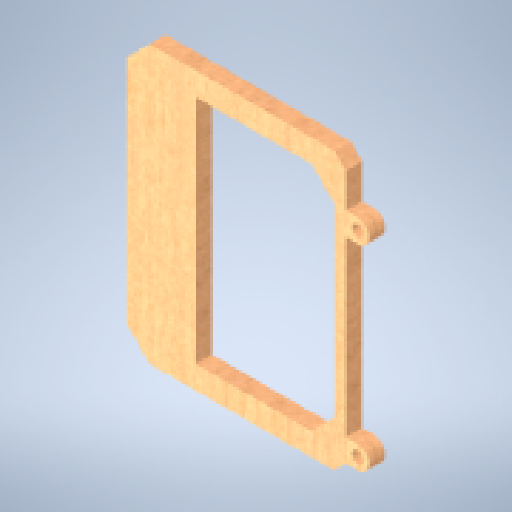
# Autodesk Inventor part: Tapa
Saved by Autodesk Inventor 2023.1 (Build 271208000, 208)
## iProperties
Created: 2022-10-30
Part Number: Tapa
Material: MDF Medium Density Fiberboard
Document SubType Name: Modeling
Designer: Daniel Peña
Density: 0.8 g/cm^3
Appearance: Cherry - Natural Low Gloss
Author: Daniel Peña
Autodesk Inventor part; units mm, degrees
ref_plane "YZ Plane" through (0, 0, 0) normal (1, 0, 0) x (0, 1, 0)
ref_plane "XZ Plane" through (0, 0, 0) normal (0, 1, 0) x (-1, 0, 0)
ref_plane "XY Plane" through (0, 0, 0) normal (0, 0, 1) x (1, 0, 0)
sketch "Sketch1" plane through (0, 0, 0) normal (0, 0, 1) x (1, 0, 0)
  circle A0 centre (47.5, -35) radius 2.5 projected
  circle A1 centre (47.5, 50) radius 2.5 projected
  circle A2 centre (47.5, 35) radius 2.5 projected
  circle A3 centre (47.5, -50) radius 2.5 projected
  line L0 (50, -65) -> (52.5, -62.5) projected
  line L1 (52.5, -62.5) -> (52.5, -15) projected
  line L2 (52.5, -15) -> (37.5, -15) projected
  line L3 (37.5, -15) -> (37.5, -40) projected
  line L4 (37.5, -40) -> (27.5, -50) projected
  line L5 (27.5, -50) -> (-22.5, -50) projected
  line L6 (-22.5, -50) -> (-22.5, 50) projected
  line L7 (-22.5, 50) -> (27.5, 50) projected
  line L8 (27.5, 50) -> (37.5, 40) projected
  line L9 (37.5, 40) -> (37.5, 15) projected
  line L10 (37.5, 15) -> (52.5, 15) projected
  line L11 (52.5, 15) -> (52.5, 62.5) projected
  line L12 (52.5, 62.5) -> (50, 65) projected
  line L13 (50, 65) -> (-52.5, 65) projected
  line L14 (-52.5, 65) -> (-52.5, -65) projected
  line L15 (-52.5, -65) -> (50, -65) projected
  line L16 (-42.5, 60) -> (37.5, 60)
  line L17 (37.5, -60) -> (-42.5, -60)
  line L18 (-52.5, -50) -> (-52.5, 50)
  line L19 (0, 0) -> (31.4372, 0) construction
  line L20 (42.5, -54.9524) -> (47.5, -54.9524)
  line L21 (52.5, -49.9524) -> (52.5, -49.9524)
  line L22 (47.5, -44.9524) -> (42.5, -44.9524)
  arc A4 (52.5, -49.9524) -> (47.5, -44.9524) centre (47.5, -49.9524) ccw
  arc A5 (47.5, -54.9524) -> (52.5, -49.9524) centre (47.5, -49.9524) ccw
  line L23 (42.5, -54.9524) -> (42.5, -55)
  line L24 (42.5, 30) -> (47.5, 30)
  line L25 (47.5, 40) -> (42.5, 40)
  arc A6 (52.5, 35) -> (47.5, 40) centre (47.5, 35) ccw
  arc A7 (47.5, 30) -> (52.5, 35) centre (47.5, 35) ccw
  line L26 (42.5, 55) -> (42.5, 40)
  line L27 (42.5, 30) -> (42.5, -44.9524)
  line L28 (-22.5, 40) -> (37.5, 40)
  line L29 (37.5, 40) -> (37.5, -40)
  line L30 (37.5, -40) -> (-22.5, -40)
  line L31 (-22.5, -40) -> (-22.5, 40)
  line L32 (-52.5, 50) -> (-42.5, 60)
  line L33 (-52.5, -50) -> (-42.5, -60)
  line L34 (37.5, 60) -> (42.5, 55)
  line L35 (37.5, -60) -> (42.5, -55)
  point P0 (-52.5, 60)
  point P1 (42.5, -60)
  point P2 (42.5, 60)
  point P3 (-52.5, -60)
  point P4 (52.5, -44.9524)
  point P5 (52.5, -54.9524)
  point P6 (-52.5, 50)
  dimension "d2" = 10
  dimension "d3" = 10
  dimension "d4" = 10
  dimension "d5" = 5
  dimension "d6" = 5
  dimension "d7" = 5
  dimension "d8" = 5
  dimension "d9" = 30
  dimension "d10" = 10
  dimension "d11" = 10
  dimension "d12" = 10
  dimension "d13" = 10
  dimension "d14" = 10
  dimension "d15" = 5
  dimension "d16" = 5
  dimension "d17" = 5
  dimension "d18" = 5
  constraints: 40 end point, 12 point on line, 8 parallel, 8 point on circle, 6 tangent, 5 horizontal, 5 perpendicular, 4 centre point, 4 collinear, 2 concentric, 2 other
  measures "d2" distance between parallel lines of L5 L17
  measures "d3" distance of L22.end point (52.5, -44.952)
  measures "d4" distance of point (52.5, -44.952) point (52.5, -54.952)
  measures "d5" radius of A4
  measures "d6" radius of A6
  measures "d7" distance of L24.start L24.end
  measures "d8" distance of L25.start L25.end
  measures "d9" distance between parallel lines of L18 L31
  measures "d10" distance between parallel lines of L7 L28
  measures "d11" distance of L18.end point (-52.5, 60)
  measures "d12" distance of L16.start point (-52.5, 60)
  measures "d13" distance of L18.start point (-52.5, -60)
  measures "d14" distance of L17.end point (-52.5, -60)
  measures "d15" distance of L16.end point (42.5, 60)
  measures "d16" distance of L26.start point (42.5, 60)
  measures "d17" distance of L17.start point (42.5, -60)
  measures "d18" distance of L23.end point (42.5, -60)
extrude "Extrusion1" add sketch "Sketch1" along normal blind 7 contours A5 L20 L23 L35 L17 L33 L14 L32 L16 L34 L26 L25 A6 A7 L24 L27 L10 L9 L8 L7 L6 L5 L4 L3 L2 L22 A4 | L2 L29 L10 L27
equation "\"d12\" = d11"
equation "\"d13\" = d11"
equation "\"d14\" = d13"
equation "\"d16\" = d15"
equation "\"d17\" = d15"
equation "\"d18\" = d17"
body "Solid1"
